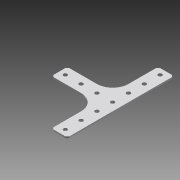
# Autodesk Inventor part: T-gusset
Saved by Autodesk Inventor 2015 (Build 190159000, 159)
## iProperties
Created: 2015-01-30
Part Number: T-gusset
Material: Generic
Document SubType Name: Sheet Metal
Designer: chapale16
Density: 1 g/cm^3
Sheet Metal Rule: Default
Appearance: Aluminum - Dark
Author: chapale16
Autodesk Inventor part; units mm, degrees
ref_plane "YZ Plane" through (0, 0, 0) normal (1, 0, 0) x (0, 1, 0)
ref_plane "XZ Plane" through (0, 0, 0) normal (0, 1, 0) x (-1, 0, 0)
ref_plane "XY Plane" through (0, 0, 0) normal (0, 0, 1) x (1, 0, 0)
sketch "Sketch1" plane through (0, 0, 0) normal (0, 1, 0) x (-1, 0, 0)
  line L0 (3.175, -3.175) -> (22.225, -3.175)
  line L1 (0, 161.925) -> (0, 0)
  line L2 (25.4, 161.925) -> (25.4, 120.65)
  line L3 (50.8, 95.25) -> (95.25, 95.25)
  line L4 (25.4, 0) -> (25.4, 44.45)
  line L5 (50.8, 69.85) -> (95.25, 69.85)
  arc A0 (25.4, 120.65) -> (50.8, 95.25) centre (50.8, 120.65) ccw
  line L6 (0, 0) -> (3.175, -3.175)
  line L7 (25.4, 0) -> (22.225, -3.175)
  arc A1 (50.8, 69.85) -> (25.4, 44.45) centre (50.8, 44.45) ccw
  line L8 (98.425, 73.025) -> (98.425, 92.075)
  line L9 (98.425, 73.025) -> (95.25, 69.85)
  line L10 (95.25, 95.25) -> (98.425, 92.075)
  line L11 (25.4, 161.925) -> (25.4, 165.1)
  line L12 (0, 161.925) -> (0, 165.1)
  line L13 (0, 165.1) -> (0, 165.1)
  line L14 (3.175, 168.275) -> (22.225, 168.275)
  line L15 (25.4, 165.1) -> (25.4, 165.1)
  line L16 (22.225, 168.275) -> (25.4, 165.1)
  line L17 (3.175, 168.275) -> (0, 165.1)
  point P0 (92.075, 69.85)
  point P1 (95.25, 69.85)
  point P2 (0, 168.275)
  point P3 (25.4, 168.275)
  dimension "d6" = 25.4
  dimension "d21" = 25.4
  dimension "d44" = 165.1
  dimension "d63" = 44.45
  dimension "d64" = 44.45
  dimension "d65" = 3.175
  dimension "d67" = 3.175
  dimension "d70" = 3.175
  dimension "d91" = 3.175
  dimension "d92" = 3.175
  dimension "d93" = 3.175
  dimension "d94" = 3.175
  constraints: 36 end point, 10 point on line, 4 point on circle, 4 tangent, 2 centre point, 2 perpendicular, 2 vertical, 1 horizontal, 1 parallel
  measures "d6" radius of A0
  measures "d21" radius of A1
  measures "d44" distance of L12.end L1.end
  measures "d63" distance of L4.start L4.end
  measures "d64" distance of L11.end L2.end
  measures "d65" distance of L2.start L11.end
  measures "d67" distance of L1.start L12.end
  measures "d70" distance of point (92.075, 69.85) point (95.25, 69.85)
  measures "d91" distance of L14.end point (25.4, 168.275)
  measures "d92" distance of L15.start point (25.4, 168.275)
  measures "d93" distance of L14.start point (0, 168.275)
  measures "d94" distance of L13.end point (0, 168.275)
extrude "Extrusion1" add sketch "Sketch1" along normal blind 2.54
hole "Hole2" at (-12.7, 2.54, 82.55) direction (0, -1, 0) diameter 6.35 end through all
pattern_linear "Rectangular Pattern4" count 4 spacing 25.4 along (-1, 0, 0) of "Hole2"
pattern_linear "Rectangular Pattern5" count 7 spacing 25.4 along (0, 0, -1) of "Hole2" first direction both ways yes
equation "\"d21\" = d6"
equation "\"d67\" = d65"
equation "\"d92\" = d91"
equation "\"d93\" = d91"
equation "\"d94\" = d93"
equation "\"d79\" = Thickness"
equation "\"BendRadius\" = Thickness"
equation "\"BendReliefWidth\" = Thickness"
equation "\"BendReliefDepth\" = 0.5 * Thickness"
equation "\"CornerReliefSize\" = 4 * Thickness"
equation "\"MinimumRemnant\" = 2 * Thickness"
equation "\"TransitionRadius\" = BendRadius"
equation "\"JacobiRadiusSize\" = BendRadius"
equation "\"GapSize\" = Thickness"
equation "\"Thickness\" = 3.048"
body "Solid1"
